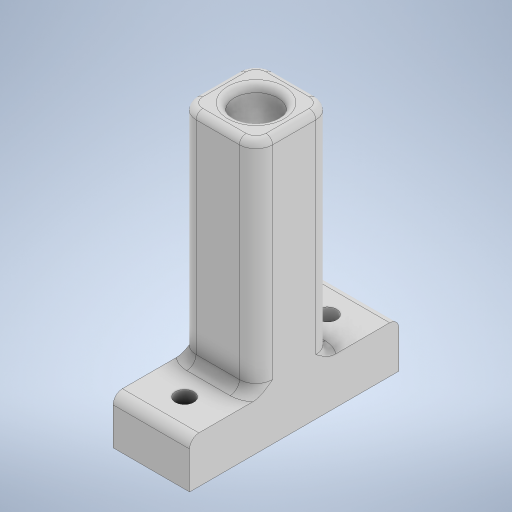
# Autodesk Inventor part: Rod Holder V1
Saved by Autodesk Inventor 2024.2 (Build 282272000, 272)
## iProperties
Created: 2024-07-26
Part Number: Rod Holder V1
Material: Generic
Document SubType Name: Modeling
Designer: balmo
Density: 1 g/cm^3
Appearance: Default
Author: balmo
## iProperties of the stored document Rod Holder V1_3DPrint.ipt
Created: 2024-08-04
Part Number: Rod Holder V1_3DPrint
Material: Generic
Document SubType Name: Modeling
Designer: balmo
Density: 1 g/cm^3
Appearance: Default
Author: balmo
Autodesk Inventor part; units mm, degrees
ref_plane "YZ Plane" through (0, 0, 0) normal (1, 0, 0) x (0, 1, 0)
ref_plane "XZ Plane" through (0, 0, 0) normal (0, 1, 0) x (-1, 0, 0)
ref_plane "XY Plane" through (0, 0, 0) normal (0, 0, 1) x (1, 0, 0)
sketch "Sketch1" plane through (0, 0, 0) normal (0, 1, 0) x (-1, 0, 0)
  circle A0 centre (0, 0) radius 4.1275
  line L0 (7.3152, 7.3152) -> (-7.3152, 7.3152)
  line L1 (-7.3152, 7.3152) -> (-7.3152, -7.3025)
  line L2 (-7.3152, -7.3025) -> (7.3152, -7.3025)
  line L3 (7.3152, -7.3025) -> (7.3152, 7.3152)
  line L4 (7.3152, 20.0152) -> (-7.3152, 20.0152)
  line L5 (-7.3152, 20.0152) -> (-7.3152, -20.0025)
  line L6 (-7.3152, -20.0025) -> (7.3152, -20.0025)
  line L7 (7.3152, -20.0025) -> (7.3152, 20.0152)
  circle A1 centre (0, 13.6652) radius 1.778
  circle A2 centre (0, -13.6525) radius 1.778
  line L8 (7.3152, 7.3152) -> (20.0152, 7.3152)
  line L9 (20.0152, 7.3152) -> (20.0152, -7.3025)
  line L10 (20.0152, -7.3025) -> (7.3152, -7.3025)
  line L11 (7.3152, -7.3025) -> (7.3152, 7.3152)
  line L12 (-7.3152, 7.3152) -> (-20.0152, 7.3152)
  line L13 (-20.0152, 7.3152) -> (-20.0152, -7.3025)
  line L14 (-20.0152, -7.3025) -> (-7.3152, -7.3025)
  line L15 (-7.3152, -7.3025) -> (-7.3152, 7.3152)
  circle A3 centre (13.6652, 0.0063) radius 1.9812
  circle A4 centre (-13.6652, 0.0063) radius 1.9812
  point P0 (-7.3152, 7.3152)
  point P1 (-7.3152, -7.3025)
  point P2 (-7.3152, -7.3025)
  dimension "d0" = 8.255
  dimension "d1" = 7.3025
  dimension "d2" = 7.3152
  dimension "d3" = 7.3152
  dimension "d4" = 7.3152
  dimension "d5" = 3.556
  dimension "d6" = 3.556
  dimension "d7" = 12.7
  dimension "d8" = 12.7
  dimension "d9" = 6.35
  dimension "d10" = 6.35
  dimension "d23" = 12.7
  dimension "d24" = 12.7
  dimension "d25" = 3.9624
  dimension "d26" = 3.9624
  constraints: 32 end point, 8 parallel, 5 centre point, 4 horizontal, 4 perpendicular, 1 coincident
  measures "d0" diameter of A0
  measures "d1" distance from line of A0.centre L2
  measures "d2" distance from line of L0 A0.centre
  measures "d3" distance from line of L3 A0.centre
  measures "d4" distance from line of A0.centre L1
  measures "d5" diameter of A1
  measures "d6" diameter of A2
  measures "d7" distance between parallel lines of L6 L2
  measures "d8" distance between parallel lines of L4 L0
  measures "d9" distance from line of L4 A1.centre
  measures "d10" distance from line of L6 A2.centre
  measures "d23" distance of L9.end L10.end
  measures "d24" distance of L14.end L13.end
  measures "d25" diameter of A3
  measures "d26" diameter of A4
extrude "Extrusion1" add sketch "Sketch1" along normal blind 8.89 contours L3 L2 L1 L0 | L0 L5 L4 L7 | L7 L6 L5 L2
extrude "Extrusion2" add sketch "Sketch1" along normal blind 50.8 contours L3 L2 L1 L0
fillet "Fillet1" radius 3.175 4 edges at (7.3152, 29.845, 7.3152) (-7.3152, 29.845, 7.3152) (7.3152, 29.845, -7.3025) (-7.3152, 29.845, -7.3025)
fillet "Fillet3" radius 1.27 1 edges at (4.1275, 50.8, 0)
extrude "Extrusion3" add sketch "Sketch1" along normal blind 31.75 contours A0
fillet "Fillet5" radius 1.778 2 edges at (0, 8.89, 20.0152) (0, 8.89, -20.0025)
fillet "Fillet6" radius 1.778 6 edges at (0, 8.89, 7.3152) (-6.3853, 8.89, 6.3853) (-6.3853, 8.89, -6.3726) (0, 8.89, -7.3025) (6.3853, 8.89, -6.3726) (6.3853, 8.89, 6.3853)
fillet "Fillet7" radius 1.27 8 edges at (6.3853, 50.8, 6.3853) (7.3152, 50.8, 0.0063) (6.3853, 50.8, -6.3726) (0, 50.8, -7.3025) (-6.3853, 50.8, -6.3726) (-7.3152, 50.8, 0.0064) (-6.3853, 50.8, 6.3853) (0, 50.8, 7.3152)
body "Solid1"
